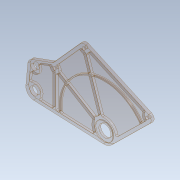
# Autodesk Inventor part: 脚フレーム外側後
Saved by Autodesk Inventor 2020.2 (Build 242310000, 310)
## iProperties
Created: 2020-03-11
Part Number: 脚フレーム外側後
Material: ポリカーボネート、スモーク
Document SubType Name: Modeling
Designer: aoyam
Density: 1.2 g/cm^3
Appearance: ポリカーボネート - スモーク
Mass: 10.0522 g
Surface Area: 149.95 cm^2
Volume: 8.37685 cm^3
Author: aoyam
Autodesk Inventor part; units mm, degrees
ref_plane "YZ Plane" through (0, 0, 0) normal (1, 0, 0) x (0, 1, 0)
ref_plane "XZ Plane" through (0, 0, 0) normal (0, 1, 0) x (-1, 0, 0)
ref_plane "XY Plane" through (0, 0, 0) normal (0, 0, 1) x (1, 0, 0)
sketch "スケッチ1" plane through (0, 0, 0) normal (0, 0, 1) x (1, 0, 0)
  circle A0 centre (73.2586, 61.8703) radius 1.5
  circle A1 centre (136.6856, 33.2211) radius 1.5
  circle A2 centre (93.6, 0) radius 9.025
  circle A3 centre (43.9613, 30) radius 1.5
  circle A4 centre (73.2586, 61.8703) radius 1.5
  circle A5 centre (136.6856, 33.2211) radius 1.5
  circle A6 centre (93.6, 0) radius 6.025
  circle A7 centre (43.9613, 30) radius 1.5
  circle A8 centre (23.2, 0) radius 4.025
  circle A9 centre (23.2, 0) radius 5
  circle A10 centre (23.2, 20.8573) radius 3
  circle A11 centre (73.2586, 61.8703) radius 4.5
  circle A12 centre (136.6856, 33.2211) radius 4.5
  circle A13 centre (43.9613, 30) radius 4.5
  circle A14 centre (23.2, 20.8573) radius 6
  circle A15 centre (23.2, 0) radius 8
  line L0 (17.2276, 21.4326) -> (15.2369, 0.7671)
  line L1 (22.8562, -7.9926) -> (94.1672, -11.0596)
  line L2 (100.9543, -8.2306) -> (139.841, 30.0127)
  line L3 (75.1109, 65.9713) -> (138.538, 37.3222)
  line L4 (21.1502, 26.4963) -> (42.424, 34.2293)
  line L5 (42.424, 34.2293) -> (69.9085, 64.8748)
  circle A16 centre (93.6, 0) radius 11.025
  line L6 (72.6754, 67.0714) -> (140.5934, 36.3938) construction
  line L7 (70.544, 65.4593) -> (72.6754, 67.0714)
  line L8 (140.5934, 36.3938) -> (141.0798, 34.1916) construction
  line L9 (56.2506, 71.8837) -> (155.5887, 40.928) construction
  line L10 (141.1856, 33.2211) -> (141.1856, 45.4163) construction
  line L11 (122.4554, 48.6344) -> (138.6856, 43.5768) construction
  line L12 (121.7116, 46.2476) -> (137.9419, 41.19) construction
  line L13 (139.4294, 45.9636) -> (123.1992, 51.0212) construction
  arc A17 (123.1992, 51.0212) -> (121.7116, 46.2476) centre (122.4554, 48.6344) ccw construction
  arc A18 (137.9419, 41.19) -> (139.4294, 45.9636) centre (138.6856, 43.5768) ccw construction
  circle A19 centre (122.4554, 48.6344) radius 1.5 construction
  circle A20 centre (138.6856, 43.5768) radius 1.5 construction
  point P0 (0, 0)
  point P1 (0, 0)
  point P2 (0, 0)
  point P3 (101.3306, -7.8606)
  point P4 (93.1263, -11.0148)
  point P5 (130.5705, 46.1056)
  point P6 (74.8601, 66.0846)
  point P7 (141.1856, 43.5768)
  dimension "d14" = 3
  dimension "d15" = 3
  dimension "d16" = 3
  dimension "d17" = 18.05
  dimension "d19" = 8.05
  dimension "d27" = 6
  dimension "d29" = 3
  dimension "d30" = 3
  dimension "d31" = 3
  dimension "d32" = 3
  dimension "d33" = 3
  dimension "d34" = 12.05
  dimension "d35" = 2
  dimension "d75" = 0
  dimension "d84" = 7
  dimension "d85" = 17
  dimension "d86" = 5
  dimension "d87" = 3
  dimension "d88" = 3
  constraints: 30 end point, 20 centre point, 19 tangent, 15 point on circle, 2 coincident, 2 collinear, 1 concentric, 1 midpoint, 1 parallel, 1 point on line, 1 vertical, 10 other
  measures "d14" diameter of A3
  measures "d15" diameter of A0
  measures "d16" diameter of A1
  measures "d17" diameter of A2
  measures "d19" diameter of A8
  measures "d27" diameter of A10
  measures "d29" radial gap between concentric circles of A0 A11
  measures "d30" radial gap between concentric circles of A1 A12
  measures "d31" diameter of A3
  measures "d32" radial gap between concentric circles of A10 A14
  measures "d33" radial gap between concentric circles of A9 A15
  measures "d34" diameter of A6
  measures "d35" radial gap between concentric circles of A16 A2
  measures "d75" distance between parallel lines of L3 L6
  measures "d84" angle of L3 L9
  measures "d85" distance of L11.start L11.end
  measures "d86" diameter of A18
  measures "d87" diameter of A19
  measures "d88" diameter of A20
extrude "押し出し4" add sketch "スケッチ1" along normal blind 3 contours A9 | A11 | A13 | A11 L3 A12 L2 A16 L1 A15 L0 A14 L4 L5 | A12 | A14 | A16 | A15
extrude "押し出し5" add sketch "スケッチ1" along normal blind 2 contours A2 | A9
sketch "スケッチ3" plane through (0, 0, 3) normal (0, 0, 1) x (1, 0, 0)
  circle A0 centre (93.6, 0) radius 9.025 projected
  line L0 (42.424, 34.2293) -> (21.1502, 26.4963) projected
  arc A1 (21.1502, 26.4963) -> (17.2276, 21.4326) centre (23.2, 20.8573) ccw projected
  line L1 (17.2276, 21.4326) -> (15.2369, 0.7671) projected
  arc A2 (15.2369, 0.7671) -> (22.8562, -7.9926) centre (23.2, 0) ccw projected
  line L2 (22.8562, -7.9926) -> (93.1263, -11.0148) projected
  arc A3 (93.1263, -11.0148) -> (101.3306, -7.8606) centre (93.6, 0) ccw projected
  line L3 (101.3306, -7.8606) -> (139.841, 30.0127) projected
  arc A4 (139.841, 30.0127) -> (138.538, 37.3222) centre (136.6856, 33.2211) ccw projected
  arc A5 (75.1109, 65.9713) -> (69.9085, 64.8748) centre (73.2586, 61.8703) ccw projected
  line L4 (69.9085, 64.8748) -> (42.424, 34.2293) projected
  circle A6 centre (23.2, 0) radius 4.025 projected
  circle A7 centre (23.2, 20.8573) radius 3 projected
  circle A8 centre (43.9613, 30) radius 1.5 projected
  circle A9 centre (73.2586, 61.8703) radius 1.5 projected
  circle A10 centre (136.6856, 33.2211) radius 1.5 projected
  circle A11 centre (93.6, 0) radius 9.025 projected
  circle A12 centre (23.2, 20.8573) radius 6
  circle A13 centre (23.2, 0) radius 7.025
  circle A14 centre (43.9613, 30) radius 4.5
  circle A15 centre (73.2586, 61.8703) radius 4.5
  circle A16 centre (136.6856, 33.2211) radius 4.5
  circle A17 centre (93.6, 0) radius 12.025
  arc A18 (23.2, 1.5) -> (23.2, -1.5) centre (23.2, 0) ccw
  arc A19 (93.6, -1.5) -> (93.6, 1.5) centre (93.6, 0) ccw
  arc A20 (93.1739, -1.4382) -> (94.0261, 1.4382) centre (93.6, 0) ccw
  arc A21 (23.6261, 22.2955) -> (22.7739, 19.4191) centre (23.2, 20.8573) ccw
  line L5 (93.6, 0) -> (43.9613, 30) construction
  line L6 (94.3759, 1.2838) -> (44.7372, 31.2838)
  line L7 (43.1854, 28.7162) -> (92.8241, -1.2838)
  arc A22 (92.8241, -1.2838) -> (94.3759, 1.2838) centre (93.6, 0) ccw
  arc A23 (44.7372, 31.2838) -> (43.1854, 28.7162) centre (43.9613, 30) ccw
  line L8 (93.6, 0) -> (73.2586, 61.8703) construction
  line L9 (95.025, 0.4685) -> (74.6835, 62.3388)
  line L10 (71.8336, 61.4018) -> (92.175, -0.4685)
  arc A24 (92.175, -0.4685) -> (95.025, 0.4685) centre (93.6, 0) ccw
  arc A25 (74.6835, 62.3388) -> (71.8336, 61.4018) centre (73.2586, 61.8703) ccw
  arc A26 (92.6841, 1.1879) -> (94.5159, -1.1879) centre (93.6, 0) ccw
  arc A27 (137.6016, 32.0332) -> (135.7697, 34.409) centre (136.6856, 33.2211) ccw
  arc A28 (21.7, 0) -> (24.7, 0) centre (23.2, 0) ccw
  arc A29 (24.7, 20.8573) -> (21.7, 20.8573) centre (23.2, 20.8573) ccw
  arc A30 (22.5955, 22.2301) -> (23.8045, 19.4845) centre (23.2, 20.8573) ccw
  arc A31 (44.5658, 28.6272) -> (43.3568, 31.3728) centre (43.9613, 30) ccw
  arc A32 (42.857, 31.0151) -> (45.0656, 28.9849) centre (43.9613, 30) ccw
  arc A33 (74.3629, 60.8551) -> (72.1543, 62.8854) centre (73.2586, 61.8703) ccw
  arc A34 (73.876, 63.2373) -> (72.6411, 60.5032) centre (73.2586, 61.8703) ccw
  arc A35 (136.0682, 31.8541) -> (137.3031, 34.5881) centre (136.6856, 33.2211) ccw
  circle A36 centre (82.2513, -6.4934) radius 1.05
  line L11 (73.876, 63.2373) -> (137.3031, 34.5881)
  arc A37 (137.7374, 32.1516) -> (137.3031, 34.5881) centre (136.6856, 33.2211) ccw
  line L12 (137.7374, 32.1516) -> (99.227, -5.7217)
  arc A38 (93.2552, -8.0176) -> (99.227, -5.7217) centre (93.6, 0) ccw
  line L13 (93.2552, -8.0176) -> (22.9852, -4.9954)
  arc A39 (18.223, 0.4794) -> (22.9852, -4.9954) centre (23.2, 0) ccw
  line L14 (18.223, 0.4794) -> (20.2138, 21.1449)
  arc A40 (22.1751, 23.6768) -> (20.2138, 21.1449) centre (23.2, 20.8573) ccw
  line L15 (22.1751, 23.6768) -> (44.1554, 31.6666)
  line L16 (44.1554, 31.6666) -> (72.1419, 62.8718)
  arc A41 (73.876, 63.2373) -> (72.1419, 62.8718) centre (73.2586, 61.8703) ccw
  circle A42 centre (30.0667, -4.249) radius 1.05
  circle A43 centre (19.9435, 7.3893) radius 1.05
  circle A44 centre (20.6093, 14.3005) radius 1.05
  circle A45 centre (28.9012, 25.0045) radius 1.05
  circle A46 centre (38.6087, 28.5331) radius 1.05
  circle A47 centre (47.7273, 34.0767) radius 1.05
  circle A48 centre (69.2302, 58.0526) radius 1.05
  circle A49 centre (78.4851, 60.0033) radius 1.05
  circle A50 centre (131.8296, 35.9083) radius 1.05
  circle A51 centre (133.0572, 29.0215) radius 1.05
  circle A52 centre (106.3757, 2.7815) radius 1.05
  line L17 (43.9613, 30) -> (43.9613, -5.8975) construction
  line L18 (42.4613, 30) -> (42.4613, -5.8975)
  line L19 (45.4613, -5.8975) -> (45.4613, 30)
  arc A53 (45.4613, 30) -> (42.4613, 30) centre (43.9613, 30) ccw
  arc A54 (42.4613, -5.8975) -> (45.4613, -5.8975) centre (43.9613, -5.8975) ccw
  circle A55 centre (93.6, 0) radius 45
  circle A56 centre (93.6, 0) radius 44
  line L20 (73.0642, 63.604) -> (137.9882, 34.2787)
  line L21 (137.9882, 34.2787) -> (138.1503, 33.5446)
  arc A57 (137.7374, 32.1516) -> (138.1503, 33.5446) centre (136.6856, 33.2211) ccw
  line L22 (137.7374, 32.1516) -> (99.227, -5.7217)
  arc A58 (93.2552, -8.0176) -> (99.227, -5.7217) centre (93.6, 0) ccw
  line L23 (93.2552, -8.0176) -> (22.9852, -4.9954)
  arc A59 (18.223, 0.4794) -> (22.9852, -4.9954) centre (23.2, 0) ccw
  line L24 (18.223, 0.4794) -> (20.2138, 21.1449)
  arc A60 (22.1751, 23.6768) -> (20.2138, 21.1449) centre (23.2, 20.8573) ccw
  line L25 (22.1751, 23.6768) -> (44.1554, 31.6666)
  line L26 (44.1554, 31.6666) -> (72.1419, 62.8718)
  arc A61 (72.3537, 63.0666) -> (72.1419, 62.8718) centre (73.2586, 61.8703) ccw
  line L27 (72.3537, 63.0666) -> (73.0642, 63.604)
  line L28 (108.616, 47.5457) -> (109.4236, 47.1809)
  line L29 (138.538, 37.3222) -> (75.1109, 65.9713) projected
  point P0 (0, 0)
  point P1 (58.4, 0)
  point P2 (68.7807, 15)
  point P3 (83.4293, 30.9351)
  point P4 (23.2, 10.4286)
  point P5 (33.5807, 25.4286)
  point P6 (58.6099, 45.9351)
  point P7 (104.9721, 47.5457)
  point P8 (76.0086, 58.3084)
  point P9 (91.2985, 11.8027)
  point P10 (48.3682, 29.0893)
  point P11 (84.1648, 7.455)
  point P12 (88.4486, 10.8657)
  point P13 (73.1587, 57.3714)
  point P14 (46.8165, 26.5218)
  point P15 (105.6121, 0.5578)
  point P16 (134.7125, 29.1768)
  point P17 (133.4366, 36.3346)
  point P18 (77.7425, 61.4908)
  point P19 (69.3092, 59.7133)
  point P20 (46.1746, 33.9181)
  point P21 (39.4615, 29.9603)
  point P22 (27.0586, 25.4519)
  point P23 (19.7156, 15.9727)
  point P24 (18.6962, 5.3913)
  point P25 (27.9152, -5.2074)
  point P26 (84.308, -7.6328)
  point P27 (20.9952, 15.2771)
  point P28 (19.5642, 14.4012)
  point P29 (18.8984, 7.4899)
  point P30 (20.367, 6.4284)
  point P31 (29.1738, -3.6965)
  point P32 (30.0216, -5.298)
  point P33 (82.2062, -7.5424)
  point P34 (83.1627, -5.9719)
  point P35 (38.25, 29.52)
  point P36 (28.5425, 25.9913)
  point P37 (28.0521, 24.3868)
  point P38 (39.6213, 28.8106)
  point P39 (68.4485, 58.7536)
  point P40 (46.9457, 34.7777)
  point P41 (47.0149, 33.3054)
  point P42 (69.9923, 58.7748)
  point P43 (107.112, 2.0328)
  point P44 (133.7934, 28.2729)
  point P45 (133.7436, 29.816)
  point P46 (132.7483, 35.3999)
  point P47 (132.2618, 36.8652)
  point P48 (78.9173, 60.9602)
  point P49 (77.4963, 60.3565)
  point P50 (105.3498, 2.5581)
  point P51 (43.9613, 12.0512)
  point P52 (45.4599, -5.962)
  point P53 (82.613, 4.8875)
  point P54 (45.4613, 25.7574)
  point P55 (42.4613, -5.833)
  point P56 (42.4613, 25.7574)
  point P57 (78.4406, 41.3061)
  point P58 (56.7408, 24.0292)
  point P59 (49.0174, -6.115)
  point P60 (54.3328, 21.9792)
  point P61 (55.1891, 21.4616)
  point P62 (50.0331, -6.1587)
  point P63 (80.978, 43.1936)
  point P64 (130.7968, 25.3258)
  point P65 (130.0719, 24.613)
  point P66 (81.2905, 42.2431)
  point P67 (55.8845, 24.5467)
  point P68 (78.1281, 42.2566)
  point P69 (75.7375, 65.6259)
  point P70 (69.3092, 59.7133)
  point P71 (77.7425, 61.4908)
  dimension "d37" = 3
  dimension "d38" = 3
  dimension "d39" = 3
  dimension "d40" = 3
  dimension "d41" = 3
  dimension "d42" = 3
  dimension "d43" = 3
  dimension "d44" = 3
  dimension "d45" = 3
  dimension "d46" = 3
  dimension "d47" = 3
  dimension "d48" = 3
  dimension "d49" = 3
  dimension "d50" = 3
  dimension "d51" = 3
  dimension "d53" = 2.1
  dimension "d59" = 2.1
  dimension "d60" = 2.1
  dimension "d61" = 2.1
  dimension "d62" = 2.1
  dimension "d64" = 2.1
  dimension "d65" = 2.1
  dimension "d66" = 2.1
  dimension "d67" = 2.1
  dimension "d68" = 2.1
  dimension "d69" = 2.1
  dimension "d70" = 2.1
  dimension "d72" = 1.5
  dimension "d73" = 90
  dimension "d74" = 1
  constraints: 60 point on circle, 54 end point, 50 centre point, 36 tangent, 7 concentric, 3 midpoint, 3 parallel, 3 point on line, 1 coincident, 1 vertical, 18 other
  measures "d37" radial gap between concentric circles of A13 A6
  measures "d38" radial gap between concentric circles of A12 A7
  measures "d39" radial gap between concentric circles of A8 A14
  measures "d40" radial gap between concentric circles of A9 A15
  measures "d41" radial gap between concentric circles of A16 A10
  measures "d42" radial gap between concentric circles of A0 A17
  measures "d43" diameter of A19
  measures "d44" diameter of A21
  measures "d45" diameter of A23
  measures "d46" diameter of A25
  measures "d47" diameter of A27
  measures "d48" diameter of A29
  measures "d49" diameter of A31
  measures "d50" diameter of A33
  measures "d51" diameter of A35
  measures "d53" diameter of A36
  measures "d59" diameter of A42
  measures "d60" diameter of A43
  measures "d61" diameter of A44
  measures "d62" diameter of A45
  measures "d64" diameter of A46
  measures "d65" diameter of A47
  measures "d66" diameter of A48
  measures "d67" diameter of A49
  measures "d68" diameter of A50
  measures "d69" diameter of A51
  measures "d70" diameter of A52
  measures "d72" radius of A54
  measures "d73" diameter of A55
  measures "d74" radial gap between concentric circles of A55 A56
fillet "フィレット4" radius 2.1 1 edges at (42.424, 34.2293, 1.5)
extrude "押し出し9" cut sketch "スケッチ3" against normal blind 2.3 contours L9 A56 L12 A52 A17 | A17 L6 A56 L10 | A52 | L9 A15 A49 L11 A50 A16 A51 L12 A55 | A17 A36 L13 A56 L7 | A36 | A55 L6 A14 A47 L16 A48 A15 L10 | A15 L11 A49 | A49 | A51 | A55 L13 A54 L19 A14 L7 | A48 | A50 | L13 A42 A13 A43 L14 A44 A12 A45 L15 A46 A14 L18 | A47 | A42 | A46 | A44 | A7 | A45 | A43
fillet "フィレット5" radius 1.05 24 edges at (46.8165, 26.5218, 1.85) (48.3682, 29.0893, 1.85) (73.1587, 57.3714, 1.85) (76.0086, 58.3084, 1.85) (84.1648, 7.455, 1.85) (88.4486, 10.8657, 1.85) (91.2985, 11.8027, 1.85) (42.4613, -5.833, 1.85) (45.4599, -5.962, 1.85) (42.4613, 25.7574, 1.85) (82.613, 4.8875, 1.85) (49.0174, -6.115, 1.85) (50.0331, -6.1587, 1.85) (55.8845, 24.5467, 1.85) (54.3328, 21.9792, 1.85) (55.1891, 21.4616, 1.85) (56.7408, 24.0292, 1.85) (78.1281, 42.2566, 1.85) (78.4406, 41.3061, 1.85) (80.978, 43.1936, 1.85) (81.2905, 42.2431, 1.85) (130.7968, 25.3258, 1.85) (130.0719, 24.613, 1.85) (77.7425, 61.4908, 1.85)
